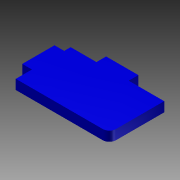
# Autodesk Inventor part: OpenROV 2.3 Dev EChassis Horz Blinder
Saved by Autodesk Inventor 2012 (Build 160160000, 160)
## iProperties
Created: 2011-12-20
Part Number: OpenROV 2.3 Dev EChassis Horz Blinder
Document SubType Name: Modeling
Designer: user
Density: 1 g/cm^3
Material: Default
Author: user
Autodesk Inventor part; units mm, degrees
ref_plane "YZ Plane" through (0, 0, 0) normal (1, 0, 0) x (0, 1, 0)
ref_plane "XZ Plane" through (0, 0, 0) normal (0, 1, 0) x (-1, 0, 0)
ref_plane "XY Plane" through (0, 0, 0) normal (0, 0, 1) x (1, 0, 0)
sketch "Sketch1" plane through (0, 0, 0) normal (0, 0, 1) x (1, 0, 0)
  line L0 (0, 0) -> (27, 0)
  line L1 (18, 17) -> (18, 20)
  line L2 (18, 20) -> (8, 20)
  line L3 (8, 20) -> (8, 17)
  line L4 (29, 17) -> (18, 17)
  line L5 (-3, 15) -> (-3, 5)
  line L6 (-3, 5) -> (0, 5)
  line L7 (0, 5) -> (0, 0)
  arc A0 (27, 0) -> (29, 2) centre (27, 2) ccw
  line L8 (-3, 15) -> (0, 15)
  line L9 (29, 17) -> (29, 2)
  line L10 (0, 15) -> (0, 17)
  line L11 (0, 17) -> (8, 17)
  point P0 (25, 0)
  dimension "d8" = 10
  dimension "d10" = 3
  dimension "d15" = 2
  dimension "d16" = 10
  dimension "d25" = 3
  dimension "d26" = 5
  dimension "d33" = 17
  dimension "d35" = 11
  dimension "d36" = 11
  dimension "d38" = 2
  dimension "d39" = 8
  dimension "d40" = 32
  dimension "d41" = 3
  constraints: 24 end point, 3 parallel, 3 perpendicular, 2 point on circle, 2 tangent, 1 centre point, 1 horizontal, 1 point on line
  measures "d8" distance of L5.start L5.end
  measures "d10" distance of L5.end L6.end
  measures "d15" radius of A0
  measures "d16" distance of L1.end L2.end
  measures "d25" distance of L1.start L1.end
  measures "d26" distance between parallel lines of L0 L6
  measures "d33" distance between parallel lines of L0 L4
  measures "d35" distance between parallel lines of L3 L5
  measures "d36" distance of L4.start L1.start
  measures "d38" distance of L8.end L10.end
  measures "d39" distance of L10.end L3.end
  measures "d40" distance between parallel lines of L9 L5
  measures "d41" distance of L2.end L3.end
extrude "Extrusion1" add sketch "Sketch1" along normal blind 3
body "Solid1"
